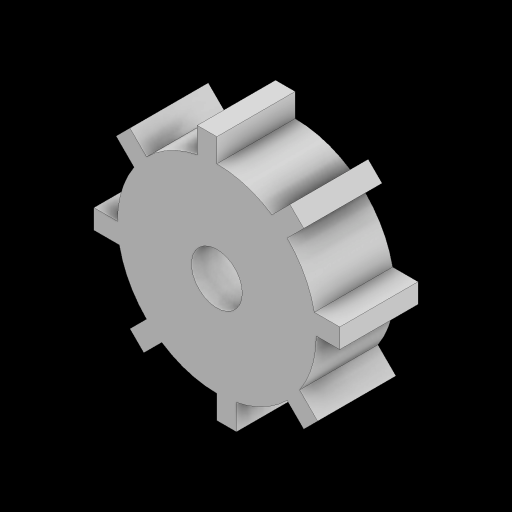
# Autodesk Inventor part: motor gear
Saved by Autodesk Inventor 2023 (Build 270158000, 158)
## iProperties
Created: 2023-07-14
Part Number: motor gear
Material: Generic
Document SubType Name: Modeling
Designer: pif12
Density: 1 g/cm^3
Appearance: Default
Author: pif12
Autodesk Inventor part; units mm, degrees
ref_plane "YZ Plane" through (0, 0, 0) normal (1, 0, 0) x (0, 1, 0)
ref_plane "XZ Plane" through (0, 0, 0) normal (0, 1, 0) x (-1, 0, 0)
ref_plane "XY Plane" through (0, 0, 0) normal (0, 0, 1) x (1, 0, 0)
sketch "Sketch1" plane through (0, 0, 0) normal (0, 0, 1) x (1, 0, 0)
  circle A0 centre (0, 0) radius 6.35
  line L0 (0, 6.35) -> (0, 7.85)
  line L1 (0, 7.85) -> (-1.25, 7.85)
  line L2 (-1.25, 7.85) -> (-1.25, 6.2258)
  line L3 (-5.5508, 5.5508) -> (-6.4347, 4.6669)
  line L4 (-6.4347, 4.6669) -> (-5.2862, 3.5184)
  line L5 (-4.4901, 4.4901) -> (-5.5508, 5.5508)
  line L6 (-7.85, 0) -> (-7.85, -1.25)
  line L7 (-7.85, -1.25) -> (-6.2258, -1.25)
  line L8 (-6.35, 0) -> (-7.85, 0)
  line L9 (-5.5508, -5.5508) -> (-4.6669, -6.4347)
  line L10 (-4.6669, -6.4347) -> (-3.5184, -5.2862)
  line L11 (-4.4901, -4.4901) -> (-5.5508, -5.5508)
  line L12 (0, -7.85) -> (1.25, -7.85)
  line L13 (1.25, -7.85) -> (1.25, -6.2258)
  line L14 (0, -6.35) -> (0, -7.85)
  line L15 (5.5508, -5.5508) -> (6.4347, -4.6669)
  line L16 (6.4347, -4.6669) -> (5.2862, -3.5184)
  line L17 (4.4901, -4.4901) -> (5.5508, -5.5508)
  line L18 (7.85, 0) -> (7.85, 1.25)
  line L19 (7.85, 1.25) -> (6.2258, 1.25)
  line L20 (6.35, 0) -> (7.85, 0)
  line L21 (5.5508, 5.5508) -> (4.6669, 6.4347)
  line L22 (4.6669, 6.4347) -> (3.5184, 5.2862)
  line L23 (4.4901, 4.4901) -> (5.5508, 5.5508)
  circle A1 centre (0, 0) radius 1.625
  point P0 (-3.5184, -5.2862)
  point P1 (4.4901, -4.4901)
  point P2 (5.2862, -3.5184)
  point P3 (6.2258, 1.25)
  point P4 (3.5184, 5.2862)
  dimension "d2" = 1.5
  dimension "d6" = 360
  dimension "d10" = 3.25
  constraints: 48 end point, 2 centre point, 2 point on circle, 1 coincident, 1 horizontal, 1 perpendicular, 1 vertical, 57 other
  measures "d2" distance of L0.start L0.end
  measures "d10" diameter of A1
extrude "Extrusion1" add sketch "Sketch1" along normal blind 5
body "Solid1"
